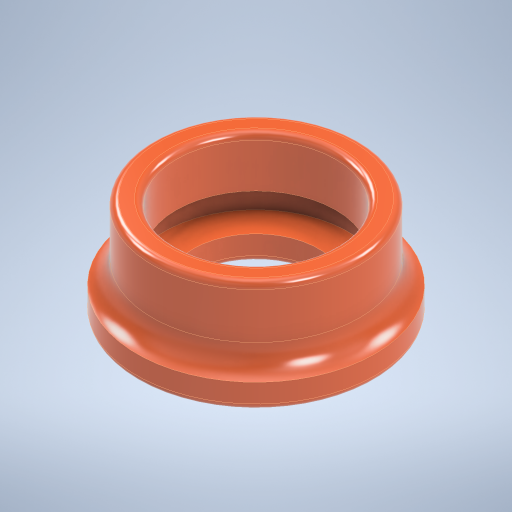
# Autodesk Inventor part: çıkçıkkarşılıkk
Saved by Autodesk Inventor 2023.2 (Build 272271000, 271)
## iProperties
Created: 2022-12-07
Part Number: çıkçıkkarşılıkk
Material: Generic
Document SubType Name: Modeling
Designer: omrfrkmll
Density: 1 g/cm^3
Appearance: Smooth - Light Orange
Author: omrfrkmll
Autodesk Inventor part; units mm, degrees
ref_plane "YZ Plane" through (0, 0, 0) normal (1, 0, 0) x (0, 1, 0)
ref_plane "XZ Plane" through (0, 0, 0) normal (0, 1, 0) x (-1, 0, 0)
ref_plane "XY Plane" through (0, 0, 0) normal (0, 0, 1) x (1, 0, 0)
sketch "Sketch1" plane through (0, 0, 0) normal (0, 0, 1) x (1, 0, 0)
  line L0 (0, 10.7366) -> (0, -7.1166)
  line L1 (0, 0) -> (9.5, 0)
  line L2 (9.5, 0) -> (9.5, 2)
  line L3 (9.5, 2) -> (8.25, 2)
  line L4 (8.25, 2) -> (8.25, 8)
  line L5 (8.25, 8) -> (6.35, 8)
  line L6 (6.35, 8) -> (6.35, 2)
  line L7 (6.35, 2) -> (0, 2)
  dimension "d0" = 19
  dimension "d1" = 12.7
  dimension "d2" = 1.9
  dimension "d3" = 2
  dimension "d6" = 6
  constraints: 16 end point, 5 perpendicular, 3 point on line, 2 vertical, 1 horizontal
  measures "d0" diameter of L2 L0
  measures "d1" diameter of L6 L0
  measures "d2" distance between parallel lines of L6 L4
  measures "d3" distance between parallel lines of L1 L7
  measures "d6" distance between parallel lines of L3 L5
revolve "Revolution1" add sketch "Sketch1" angle 360 about axis through (0, 10.7366, 0) along (0, -1, 0)
sketch "Sketch2" plane through (0, 0, 0) normal (0, 0, 1) x (1, 0, 0)
  line L0 (6.1122, 2) -> (7.35, 2)
  line L1 (8.25, 8) -> (8.25, 2)
  line L2 (7.35, 4) -> (6.1122, 4)
  line L3 (6.1122, 4) -> (6.1122, 2)
  line L4 (8.25, 3) -> (8.25, 4)
  line L5 (-8.25, 8) -> (8.25, 8) projected
  line L6 (0, 5.3477) -> (0, 2.8187)
  line L7 (7.35, 4) -> (7.35, 2)
  point P0 (0, 0)
  dimension "d7" = 4
  dimension "d8" = 2
  dimension "d9" = 14.7
  constraints: 14 end point, 4 vertical, 2 horizontal, 1 perpendicular, 1 point on line
  measures "d7" distance between parallel lines of L5 L2
  measures "d8" distance between parallel lines of L0 L2
  measures "d9" diameter of L7 L6
revolve "Revolution2" cut sketch "Sketch2" angle 360 about axis through (0, 5.3477, 0) along (0, -1, 0)
sketch "Sketch3" plane through (0, 0, 0) normal (0, -1, 0) x (1, 0, 0)
  circle A0 centre (0, 0) radius 5
  dimension "d11" = 10
  constraints: 1 centre point, 1 coincident
  measures "d11" diameter of A0
extrude "Extrusion1" cut sketch "Sketch3" against normal up to surface (2 mm away)
fillet "Fillet1" radius 2 1 edges at (-8.25, 2, 0)
fillet "Fillet2" radius 0.5 2 edges at (-6.35, 8, 0) (-8.25, 8, 0)
fillet "Fillet3" radius 0.5 2 edges at (-9.5, 0, 0) (-5, 0, 0)
body "Solid1"
